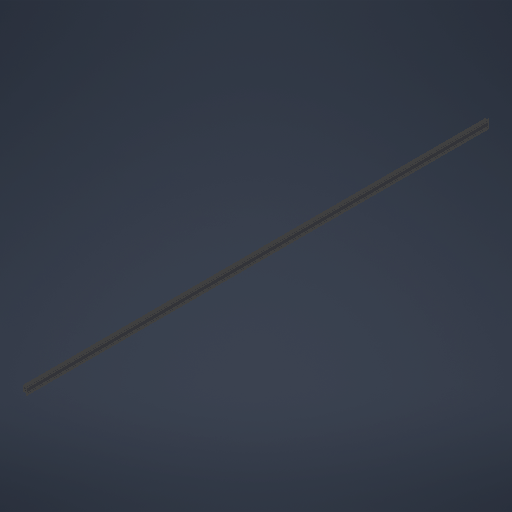
# Autodesk Inventor part: PLANTILLA SP40-04A TRAVESAÑO CENTRAL
Saved by Autodesk Inventor 2025 (Build 290162000, 162)
## iProperties
Created: 2026-01-20
Part Number: PLANTILLA SP40-04A TRAVESAÑO CENTRAL
Material: Aluminio
Document SubType Name: Modeling
Designer: ROLANDO
Density: 2.7 g/cm^3
Appearance: Satinado
Author: ROLANDO
Autodesk Inventor part; units mm, degrees
ref_plane "YZ Plane" through (0, 0, 0) normal (1, 0, 0) x (0, 1, 0)
ref_plane "XZ Plane" through (0, 0, 0) normal (0, 1, 0) x (-1, 0, 0)
ref_plane "XY Plane" through (0, 0, 0) normal (0, 0, 1) x (1, 0, 0)
sketch "Boceto1" plane through (0, 0, 0) normal (0, 0, 1) x (1, 0, 0)
  line L0 (-1.1139, -2.6665) -> (15.7105, -2.6665)
  line L1 (16.2861, -3.2421) -> (16.2861, -16.3665)
  line L2 (16.2861, -16.3665) -> (12.4861, -16.3665)
  line L3 (12.4861, -16.3665) -> (12.4861, -18.0065)
  line L4 (13.1802, -19.0165) -> (13.8861, -19.0165)
  line L5 (13.8861, -19.0165) -> (13.8861, -17.7665)
  line L6 (13.8861, -17.7665) -> (16.2861, -17.7665)
  line L7 (16.2861, -17.7665) -> (16.2861, -24.2665)
  line L8 (16.2861, -24.2665) -> (13.8861, -24.2665)
  line L9 (13.8861, -24.2665) -> (13.8861, -23.0165)
  line L10 (13.8861, -23.0165) -> (13.1802, -23.0165)
  line L11 (12.4861, -24.0265) -> (12.4861, -25.6665)
  line L12 (12.4861, -25.6665) -> (17.6861, -25.6665)
  line L13 (17.6861, -25.6665) -> (17.6861, 20.5335)
  line L14 (16.2861, -0.6909) -> (16.2861, 20.5335)
  line L15 (7.3361, 2.6189) -> (7.3361, -2.6665) construction
  arc A0 (6.2361, 3.2888) -> (8.4361, 3.2888) centre (7.3361, 1.3835) ccw
  line L16 (4.9491, 1.1335) -> (5.1503, 1.1335)
  line L17 (4.9491, 1.6335) -> (5.1503, 1.6335)
  line L18 (10.9772, -1.2665) -> (15.7105, -1.2665)
  line L19 (9.723, 1.1335) -> (9.5218, 1.1335)
  line L20 (9.723, 1.6335) -> (9.5218, 1.6335)
  line L21 (7.5861, -1.0034) -> (7.5861, -0.8022)
  line L22 (7.0861, -1.0034) -> (7.0861, -0.8022)
  arc A1 (7.0861, -1.0034) -> (7.5861, -1.0034) centre (7.3361, 1.3835) ccw
  arc A2 (9.723, 1.1335) -> (9.723, 1.6335) centre (7.3361, 1.3835) ccw
  arc A3 (4.9491, 1.6335) -> (4.9491, 1.1335) centre (7.3361, 1.3835) ccw
  circle A4 centre (7.3361, 1.3835) radius 2.4 construction
  line L23 (6.2361, 4.8271) -> (6.2361, 3.2888)
  line L24 (8.4361, 4.8271) -> (8.4361, 3.2888)
  arc A5 (10.4771, -0.406) -> (8.4361, 4.8271) centre (7.3361, 1.3835) ccw
  arc A6 (6.2361, 4.8271) -> (4.2085, -0.4294) centre (7.3361, 1.3835) ccw
  line L25 (12.4861, -18.0065) -> (13.1802, -19.0165)
  line L26 (12.4861, -24.0265) -> (13.1802, -23.0165)
  arc A7 (15.7105, -1.2665) -> (16.2861, -0.6909) centre (15.7105, -0.6909) ccw
  arc A8 (16.2861, -3.2421) -> (15.7105, -2.6665) centre (15.7105, -3.2421) ccw
  arc A9 (3.8851, -1.2665) -> (4.2085, -0.4294) centre (3.7105, -0.718) ccw
  arc A10 (10.4771, -0.406) -> (10.9772, -1.2665) centre (10.9772, -0.6909) ccw
  line L27 (-26.537, 20.5335) -> (21.9694, 20.5335) construction
  line L28 (-1.6139, -3.1665) -> (-1.6139, -7.0665)
  line L29 (-1.6139, -7.0665) -> (-4.0139, -7.0665)
  line L30 (-5.0139, -5.6665) -> (-3.5139, -5.6665)
  line L31 (-3.0139, -5.1665) -> (-3.0139, -3.1665)
  line L32 (-3.5139, -2.6665) -> (-20.7139, -2.6665)
  line L33 (-21.2139, -3.1665) -> (-21.2139, -5.1665)
  line L34 (-20.7139, -5.6665) -> (-19.2139, -5.6665)
  line L35 (-20.2139, -7.0665) -> (-22.6139, -7.0665)
  line L36 (3.8851, -1.2665) -> (-20.7139, -1.2665)
  line L37 (-21.2139, -0.7665) -> (-21.2139, 20.5335)
  line L38 (-22.6139, -7.0665) -> (-22.6139, 20.5335)
  line L39 (-19.2139, -5.6665) -> (-19.2139, -6.2653)
  line L40 (-19.2139, -6.2653) -> (-20.2139, -7.0665)
  line L41 (-5.0139, -5.6665) -> (-5.0139, -6.2653)
  line L42 (-5.0139, -6.2653) -> (-4.0139, -7.0665)
  line L43 (4.3997, 1.3835) -> (10.1666, 1.3835) construction
  arc A11 (-1.1139, -2.6665) -> (-1.6139, -3.1665) centre (-1.1139, -3.1665) ccw
  arc A12 (-3.0139, -3.1665) -> (-3.5139, -2.6665) centre (-3.5139, -3.1665) ccw
  arc A13 (-3.5139, -5.6665) -> (-3.0139, -5.1665) centre (-3.5139, -5.1665) ccw
  arc A14 (-20.7139, -2.6665) -> (-21.2139, -3.1665) centre (-20.7139, -3.1665) ccw
  arc A15 (-21.2139, -5.1665) -> (-20.7139, -5.6665) centre (-20.7139, -5.1665) ccw
  arc A16 (-21.2139, -0.7665) -> (-20.7139, -1.2665) centre (-20.7139, -0.7665) ccw
  line L44 (-1.1139, 43.7335) -> (15.7105, 43.7335)
  line L45 (16.2861, 44.3091) -> (16.2861, 57.4335)
  line L46 (16.2861, 57.4335) -> (12.4861, 57.4335)
  line L47 (12.4861, 57.4335) -> (12.4861, 59.0735)
  line L48 (13.1802, 60.0835) -> (13.8861, 60.0835)
  line L49 (13.8861, 60.0835) -> (13.8861, 58.8335)
  line L50 (13.8861, 58.8335) -> (16.2861, 58.8335)
  line L51 (16.2861, 58.8335) -> (16.2861, 65.3335)
  line L52 (16.2861, 65.3335) -> (13.8861, 65.3335)
  line L53 (13.8861, 65.3335) -> (13.8861, 64.0835)
  line L54 (13.8861, 64.0835) -> (13.1802, 64.0835)
  line L55 (12.4861, 65.0935) -> (12.4861, 66.7335)
  line L56 (12.4861, 66.7335) -> (17.6861, 66.7335)
  line L57 (17.6861, 66.7335) -> (17.6861, 20.5335)
  line L58 (16.2861, 41.7579) -> (16.2861, 20.5335)
  line L59 (7.3361, 38.4481) -> (7.3361, 43.7335) construction
  arc A17 (8.4361, 37.7782) -> (6.2361, 37.7782) centre (7.3361, 39.6835) ccw
  line L60 (4.9491, 39.9335) -> (5.1503, 39.9335)
  line L61 (4.9491, 39.4335) -> (5.1503, 39.4335)
  line L62 (10.9772, 42.3335) -> (15.7105, 42.3335)
  line L63 (9.723, 39.9335) -> (9.5218, 39.9335)
  line L64 (9.723, 39.4335) -> (9.5218, 39.4335)
  line L65 (7.5861, 42.0704) -> (7.5861, 41.8692)
  line L66 (7.0861, 42.0704) -> (7.0861, 41.8692)
  arc A18 (7.5861, 42.0704) -> (7.0861, 42.0704) centre (7.3361, 39.6835) ccw
  arc A19 (9.723, 39.4335) -> (9.723, 39.9335) centre (7.3361, 39.6835) ccw
  arc A20 (4.9491, 39.9335) -> (4.9491, 39.4335) centre (7.3361, 39.6835) ccw
  circle A21 centre (7.3361, 39.6835) radius 2.4 construction
  line L67 (6.2361, 36.2399) -> (6.2361, 37.7782)
  line L68 (8.4361, 36.2399) -> (8.4361, 37.7782)
  arc A22 (8.4361, 36.2399) -> (10.4771, 41.473) centre (7.3361, 39.6835) ccw
  arc A23 (4.2085, 41.4964) -> (6.2361, 36.2399) centre (7.3361, 39.6835) ccw
  line L69 (12.4861, 59.0735) -> (13.1802, 60.0835)
  line L70 (12.4861, 65.0935) -> (13.1802, 64.0835)
  arc A24 (16.2861, 41.7579) -> (15.7105, 42.3335) centre (15.7105, 41.7579) ccw
  arc A25 (15.7105, 43.7335) -> (16.2861, 44.3091) centre (15.7105, 44.3091) ccw
  arc A26 (4.2085, 41.4964) -> (3.8851, 42.3335) centre (3.7105, 41.785) ccw
  arc A27 (10.9772, 42.3335) -> (10.4771, 41.473) centre (10.9772, 41.7579) ccw
  line L71 (-1.6139, 44.2335) -> (-1.6139, 48.1335)
  line L72 (-1.6139, 48.1335) -> (-4.0139, 48.1335)
  line L73 (-5.0139, 46.7335) -> (-3.5139, 46.7335)
  line L74 (-3.0139, 46.2335) -> (-3.0139, 44.2335)
  line L75 (-3.5139, 43.7335) -> (-20.7139, 43.7335)
  line L76 (-21.2139, 44.2335) -> (-21.2139, 46.2335)
  line L77 (-20.7139, 46.7335) -> (-19.2139, 46.7335)
  line L78 (-20.2139, 48.1335) -> (-22.6139, 48.1335)
  line L79 (3.8851, 42.3335) -> (-20.7139, 42.3335)
  line L80 (-21.2139, 41.8335) -> (-21.2139, 20.5335)
  line L81 (-22.6139, 48.1335) -> (-22.6139, 20.5335)
  line L82 (-19.2139, 46.7335) -> (-19.2139, 47.3323)
  line L83 (-19.2139, 47.3323) -> (-20.2139, 48.1335)
  line L84 (-5.0139, 46.7335) -> (-5.0139, 47.3323)
  line L85 (-5.0139, 47.3323) -> (-4.0139, 48.1335)
  line L86 (4.3997, 39.6835) -> (10.1666, 39.6835) construction
  arc A28 (-1.6139, 44.2335) -> (-1.1139, 43.7335) centre (-1.1139, 44.2335) ccw
  arc A29 (-3.5139, 43.7335) -> (-3.0139, 44.2335) centre (-3.5139, 44.2335) ccw
  arc A30 (-3.0139, 46.2335) -> (-3.5139, 46.7335) centre (-3.5139, 46.2335) ccw
  arc A31 (-21.2139, 44.2335) -> (-20.7139, 43.7335) centre (-20.7139, 44.2335) ccw
  arc A32 (-20.7139, 46.7335) -> (-21.2139, 46.2335) centre (-20.7139, 46.2335) ccw
  arc A33 (-20.7139, 42.3335) -> (-21.2139, 41.8335) centre (-20.7139, 41.8335) ccw
  point P0 (4.8546, -1.2453)
  point P1 (9.7949, -1.2665)
  point P2 (7.2983, -2.6665)
  point P3 (16.2861, -21.0165)
  point P4 (5.0497, 1.6335)
  point P5 (9.6224, 1.6335)
  point P6 (4.8546, 42.3123)
  point P7 (9.7949, 42.3335)
  point P8 (7.2983, 43.7335)
  point P9 (16.2861, 62.0835)
  point P10 (5.0497, 39.4335)
  point P11 (9.6224, 39.4335)
  dimension "d3" = 1.4
  dimension "d4" = 1.4
  dimension "d5" = 1.4
  dimension "d6" = 1.4
  dimension "d7" = 1.4
  dimension "d8" = 1.4
  dimension "d9" = 1.4
  dimension "d12" = 4.4
  dimension "d19" = 0.5
  dimension "d22" = 4.05
  dimension "d26" = 0.5
  dimension "d30" = 0.5
  dimension "d32" = 4.8
  dimension "d35" = 1.1
  dimension "d36" = 2.2
  dimension "d37" = 1.415
  dimension "d38" = 1.415
  dimension "d39" = 0.2
  dimension "d40" = 0.2
  dimension "d43" = 23
  dimension "d44" = 4
  dimension "d45" = 9.3
  dimension "d46" = 6.5
  dimension "d50" = 5.2
  dimension "d53" = 0.2
  dimension "d55" = 0.2
  dimension "d56" = 0.25
  dimension "d57" = 0.2
  dimension "d58" = 1.4
  dimension "d66" = 2
  dimension "d67" = 2
  dimension "d68" = 2.4
  dimension "d69" = 3.01
  dimension "d70" = 6.02
  dimension "d71" = 34.5
  dimension "d72" = 111
  dimension "d74" = 0.7058
  dimension "d75" = 0.7058
  dimension "d90" = 46.2
  dimension "d91" = 1.4
  dimension "d92" = 1.4
  dimension "d93" = 1.4
  dimension "d94" = 1.4
  dimension "d96" = 3
  dimension "d97" = 14.2
  dimension "d98" = 18.2
  dimension "d99" = 21
  dimension "d100" = 40.3
  dimension "d101" = 10.35
  dimension "d102" = 0.25
  dimension "d103" = 0.25
  dimension "d104" = 27.6
  dimension "d105" = 3.4
  dimension "d106" = 3.4
  dimension "d107" = 1
  dimension "d108" = 38.7
  dimension "d109" = 38.7
  dimension "d118" = 0.5
  dimension "d119" = 92.4
  dimension "d120" = 46.4
  dimension "d121" = 55.2
  dimension "d122" = 43.6
  constraints: 174 end point, 82 symmetric about line, 80 point on circle, 34 centre point, 19 tangent, 18 point on line, 17 perpendicular, 8 equal radius, 6 coincident, 6 collinear, 6 horizontal, 6 parallel, 6 vertical, 4 midpoint, 2 equal length, 17 other
  measures "d3" distance between parallel lines of L13 L14
  measures "d4" distance between parallel lines of L13 L1
  measures "d5" distance between parallel lines of L13 L7
  measures "d6" distance between parallel lines of L12 L8
  measures "d7" distance between parallel lines of L2 L6
  measures "d8" distance between parallel lines of L3 L5
  measures "d9" distance between parallel lines of L11 L9
  measures "d12" diameter of A0
  measures "d19" distance between parallel lines of L16 L17
  measures "d22" distance from line of A5.centre L0
  measures "d26" distance between parallel lines of L19 L20
  measures "d30" distance between parallel lines of L22 L21
  measures "d32" diameter of A4
  measures "d35" distance between parallel lines of L15 L23
  measures "d36" distance between parallel lines of L24 L23
  measures "d37" radial gap between concentric circles of A0 A5
  measures "d38" radial gap between concentric circles of A6 A0
  measures "d39" radial gap between concentric circles of A4 A0
  measures "d40" radial gap between concentric circles of A4 A0
  measures "d43" distance between parallel lines of L12 L0
  measures "d44" distance between parallel lines of L10 L4
  measures "d45" distance between parallel lines of L12 L2
  measures "d46" distance between parallel lines of L8 L6
  measures "d50" distance between parallel lines of L13 L11
  measures "d53" radial gap between concentric circles of A0 A3
  measures "d55" radial gap between concentric circles of A1 A0
  measures "d56" distance between parallel lines of L21 L15
  measures "d57" radial gap between concentric circles of A2 A0
  measures "d58" distance between parallel lines of L0 L18
  measures "d66" distance from line of point (16.286, -21.017) L4
  measures "d67" distance from line of point (16.286, -21.017) L10
  measures "d68" distance between parallel lines of L7 L5
  measures "d69" vertical distance of point (16.286, -21.017) L3.end
  measures "d70" distance of L3.end L11.start
  measures "d71" angle of L5 L25
  measures "d72" angle of L26 L25
  measures "d74" distance of L4.start L4.end
  measures "d75" distance of L9.end L10.end
  measures "d90" distance between parallel lines of L12 L27
  measures "d91" distance between parallel lines of L38 L37
  measures "d92" distance between parallel lines of L32 L36
  measures "d93" distance between parallel lines of L28 L31
  measures "d94" distance between parallel lines of L29 L30
  measures "d96" distance between parallel lines of L30 L32
  measures "d97" distance between parallel lines of L41 L39
  measures "d98" distance between parallel lines of L31 L33
  measures "d99" distance between parallel lines of L38 L28
  measures "d100" distance between parallel lines of L13 L38
  measures "d101" distance from line of L13 A0.centre
  measures "d102" distance from line of point (5.05, 1.633) L43
  measures "d103" distance from line of point (9.622, 1.633) L43
  measures "d104" distance between parallel lines of L35 L27
  measures "d105" distance between parallel lines of L28 L41
  measures "d106" distance between parallel lines of L39 L38
  measures "d107" horizontal distance of L41.end L29.end
  measures "d108" angle of L29 L42
  measures "d109" angle of L35 L40
  measures "d118" radius of A11
  measures "d119" distance between parallel lines of L12 L56
  measures "d120" distance between parallel lines of L75 L32
  measures "d121" distance between parallel lines of L35 L78
  measures "d122" distance between parallel lines of L36 L79
extrude "Extrusión1" add sketch "Boceto1" against normal blind 5000
